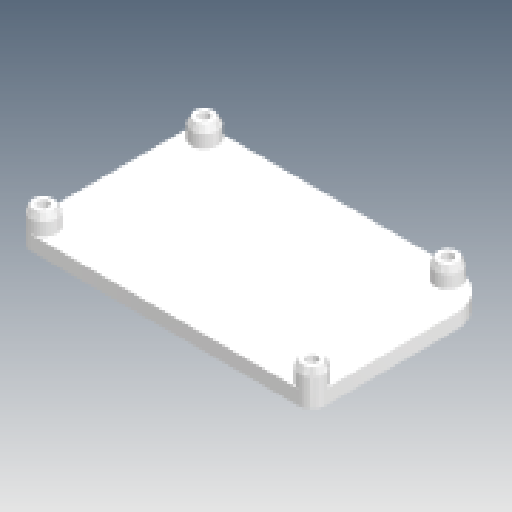
# Autodesk Inventor part: arduino_mega_standoffs_plate
Saved by Autodesk Inventor 2025.4 (Build 294407020, 407B)
## iProperties
Created: 2026-06-20
Part Number: arduino_mega_standoffs_plate
Material: Generic
Document SubType Name: Modeling
Designer: Aiden
Density: 1 g/cm^3
Appearance: Default
Author: Aiden
Autodesk Inventor part; units mm, degrees
ref_plane "YZ Plane" through (0, 0, 0) normal (1, 0, 0) x (0, 1, 0)
ref_plane "XZ Plane" through (0, 0, 0) normal (0, 1, 0) x (-1, 0, 0)
ref_plane "XY Plane" through (0, 0, 0) normal (0, 0, 1) x (1, 0, 0)
sketch "Arduino Hole Layout" plane through (0, 0, 0) normal (0, 1, 0) x (-1, 0, 0)
  circle A0 centre (43.0199, -7.0958) radius 1.55 construction
  circle A1 centre (-31.8801, -7.0958) radius 1.55 construction
  circle A2 centre (44.3199, 41.1042) radius 1.55 construction
  circle A3 centre (-38.2801, 41.1042) radius 1.55 construction
  line L0 (58.8879, -10.055) -> (-40.7911, -10.055) construction
  line L1 (-40.7911, -10.055) -> (-40.7911, 44.0634) construction
  line L2 (-40.7911, 44.0634) -> (58.8879, 44.0634) construction
  line L3 (58.8879, 44.0634) -> (58.8879, -10.055) construction
  line L4 (43.0199, -7.0958) -> (43.0199, -10.055) construction
  line L5 (44.3199, 41.1042) -> (44.3199, 44.0634) construction
  dimension "d0" = 3.1
  dimension "d1" = 74.9
  dimension "d2" = 1.3
  dimension "d3" = 48.2
  dimension "d5" = 82.6
  dimension "d9" = 15.868
  dimension "d10" = 54.1184
  dimension "d11" = 99.679
  constraints: 12 end point, 4 centre point, 4 coincident, 3 equal radius, 3 parallel, 3 perpendicular, 2 horizontal alignment, 2 point on line, 1 horizontal
  measures "d0" diameter of A0
  measures "d1" distance of A1.centre L4.start
  measures "d2" horizontal distance of L5.start L4.start
  measures "d3" vertical distance of L4.start L5.start
  measures "d5" distance of A3.centre L5.start
  measures "d9" distance from line of L3 L4.start
  measures "d10" distance of L2.end L0.start
  measures "d11" distance of L1.end L2.end
sketch "Sketch13" plane through (0, 0, 0) normal (0, 1, 0) x (-1, 0, 0)
  circle A0 centre (43.0199, -7.0958) radius 1.55 construction
  circle A1 centre (43.0199, -7.0958) radius 4
  point P0 (0, 0)
  point P1 (-38.2801, 41.1042)
  point P2 (-31.8801, -7.0958)
  point P3 (-38.2801, 41.1042)
  point P4 (44.3199, 41.1042)
  dimension "d48" = 8
  constraints: 1 centre point, 1 coincident
  measures "d48" diameter of A1
extrude "Extrusion10" add sketch "Sketch13" along normal blind 6
sketch "Sketch14" plane through (-43.0199, 6, -7.0958) normal (0, 1, 0) x (1, 0, 0)
  circle A0 centre (0, 0) radius 4 construction
  point P0 (43.0199, -7.0958)
  point P1 (81.3, -48.2)
  point P2 (-1.3, -48.2)
  point P3 (74.9, 0)
  point P4 (81.3, -48.2)
  point P5 (-1.3, -48.2)
  constraints: 3 coincident
hole "Hole2" at (-43.0199, 6, -7.0958) direction (0, -1, 0) diameter 3.25 depth 5 tip angle 118
chamfer "Chamfer2" distance 1 distance2 2 1 edges at (-39.0199, 6, -7.0958) measured on face at (-46.1856, 6, -7.4802)
pattern_sketch "Sketch Driven Pattern1" from (-43.0199, 0, -7.0958) copies at (-44.3199, 0, 41.1042) at (31.8801, 0, -7.0958) at (38.2801, 0, 41.1042)
sketch "Sketch16" plane through (-44.3199, 0, 41.1042) normal (0, -1, 0) x (1, 0, 0)
  line L0 (-4, 4) -> (86.6, 4)
  line L1 (86.6, 4) -> (86.6, -52.2)
  line L2 (86.6, -52.2) -> (-4, -52.2)
  line L3 (-4, -52.2) -> (-4, 4)
  circle A0 centre (0, 0) radius 4 projected
  circle A1 centre (82.6, 0) radius 4 projected
  circle A2 centre (1.3, -48.2) radius 4 projected
  arc A3 (-4, -46.9) -> (1.3, -52.2) centre (1.3, -46.9) ccw
  arc A4 (73.0608, -52.2) -> (86.6, -40.521) centre (74.7932, -40.521) ccw
  circle A5 centre (76.2, -48.2) radius 4 projected
  point P0 (44.3199, -41.1042)
  point P1 (76.9208, -52.1345)
  point P2 (86.6, 0)
  point P3 (82.6, 4)
  point P4 (0, 4)
  point P5 (-4, 0)
  point P6 (76.2, -52.2)
  constraints: 8 end point, 5 tangent, 4 point on circle, 4 point on line, 2 centre point, 2 horizontal, 2 parallel, 1 perpendicular, 1 vertical alignment, 4 other
extrude "Extrusion12" add sketch "Sketch16" along normal blind 4.5 contours A2 | L0 A1 L1 A4 A5 L2 A3 L3 A0 | A0 | A1 | A5
body "Solid3"
